Autodesk Fusion 360 part; units mm, degrees
(part 2 of 2)
sketch "Sketch2" plane through (0, 0, 0) normal (0, 1, 0) x (1, 0, 0) in component "Component"
  circle A0 centre (36.4389, -36.7557) radius 32
  line L0 (34.5722, -68.7012) -> (34.5722, -70.4968)
  line L1 (34.5722, -70.4968) -> (36, -73)
  line L2 (36, -73) -> (37, -73)
  line L3 (37, -73) -> (38.5721, -70.4968)
  line L4 (38.5721, -70.4968) -> (38.5721, -68.6845)
  line L5 (43.8241, -69.7477) -> (43.5406, -67.9577)
  line L6 (42.6629, -72.466) -> (43.8241, -69.7477)
  line L7 (41.6753, -72.6224) -> (42.6629, -72.466)
  line L8 (39.8735, -70.3734) -> (41.6753, -72.6224)
  line L9 (39.5926, -68.5999) -> (39.8735, -70.3734)
  line L10 (48.8943, -68.1862) -> (48.3343, -66.4626)
  line L11 (48.1726, -71.0527) -> (48.8943, -68.1862)
  line L12 (47.2216, -71.3617) -> (48.1726, -71.0527)
  line L13 (45.0902, -69.4223) -> (47.2216, -71.3617)
  line L14 (44.5353, -67.7145) -> (45.0902, -69.4223)
  line L15 (53.6578, -65.8508) -> (52.835, -64.236)
  line L16 (53.3934, -68.7949) -> (53.6578, -65.8508)
  line L17 (52.5024, -69.2489) -> (53.3934, -68.7949)
  line L18 (50.0938, -67.6667) -> (52.5024, -69.2489)
  line L19 (49.2786, -66.0668) -> (50.0938, -67.6667)
  line L20 (57.9972, -62.799) -> (56.932, -61.3328)
  line L21 (58.1967, -65.7481) -> (57.9972, -62.799)
  line L22 (57.3877, -66.3359) -> (58.1967, -65.7481)
  line L23 (54.7613, -65.15) -> (57.3877, -66.3359)
  line L24 (53.7058, -63.6974) -> (54.7613, -65.15)
  line L25 (61.8059, -59.1059) -> (60.5244, -57.8244)
  line L26 (62.4642, -61.9875) -> (61.8059, -59.1059)
  line L27 (61.7571, -62.6946) -> (62.4642, -61.9875)
  line L28 (58.9775, -61.9342) -> (61.7571, -62.6946)
  line L29 (57.7078, -60.6645) -> (58.9775, -61.9342)
  line L30 (64.9899, -54.8624) -> (63.5237, -53.7972)
  line L31 (66.0909, -57.6056) -> (64.9899, -54.8624)
  line L32 (65.5031, -58.4146) -> (66.0909, -57.6056)
  line L33 (62.6388, -58.0984) -> (65.5031, -58.4146)
  line L34 (61.1862, -57.043) -> (62.6388, -58.0984)
  line L35 (67.4709, -50.1731) -> (65.8561, -49.3504)
  line L36 (68.9875, -52.7103) -> (67.4709, -50.1731)
  line L37 (68.5335, -53.6013) -> (68.9875, -52.7103)
  line L38 (65.655, -53.7371) -> (68.5335, -53.6013)
  line L39 (64.0551, -52.9219) -> (65.655, -53.7371)
  line L40 (69.1878, -45.1535) -> (67.4642, -44.5934)
  line L41 (71.0826, -47.4222) -> (69.1878, -45.1535)
  line L42 (70.7736, -48.3732) -> (71.0826, -47.4222)
  line L43 (67.9518, -48.9576) -> (70.7736, -48.3732)
  line L44 (66.244, -48.4027) -> (67.9518, -48.9576)
  line L45 (70.0983, -39.927) -> (68.3083, -39.6435)
  line L46 (72.3247, -41.8714) -> (70.0983, -39.927)
  line L47 (72.1683, -42.859) -> (72.3247, -41.8714)
  line L48 (69.4726, -43.8777) -> (72.1683, -42.859)
  line L49 (67.6991, -43.5968) -> (69.4726, -43.8777)
  line L50 (70.18, -34.6225) -> (68.3677, -34.6225)
  line L51 (72.6831, -36.1946) -> (70.18, -34.6225)
  line L52 (72.6831, -37.1946) -> (72.6831, -36.1946)
  line L53 (70.18, -38.6224) -> (72.6831, -37.1946)
  line L54 (68.3844, -38.6224) -> (70.18, -38.6224)
  line L55 (69.4309, -29.3705) -> (67.6409, -29.654)
  line L56 (72.1491, -30.5317) -> (69.4309, -29.3705)
  line L57 (72.3056, -31.5193) -> (72.1491, -30.5317)
  line L58 (70.0566, -33.3211) -> (72.3056, -31.5193)
  line L59 (68.2831, -33.602) -> (70.0566, -33.3211)
  line L60 (67.8694, -24.3003) -> (66.1458, -24.8603)
  line L61 (70.7358, -25.022) -> (67.8694, -24.3003)
  line L62 (71.0448, -25.973) -> (70.7358, -25.022)
  line L63 (69.1054, -28.1044) -> (71.0448, -25.973)
  line L64 (67.3977, -28.6593) -> (69.1054, -28.1044)
  line L65 (65.5339, -19.5368) -> (63.9192, -20.3596)
  line L66 (68.478, -19.8012) -> (65.5339, -19.5368)
  line L67 (68.932, -20.6922) -> (68.478, -19.8012)
  line L68 (67.3499, -23.1008) -> (68.932, -20.6922)
  line L69 (65.75, -23.916) -> (67.3499, -23.1008)
  line L70 (62.4821, -15.1974) -> (61.0159, -16.2626)
  line L71 (65.4313, -14.9979) -> (62.4821, -15.1974)
  line L72 (66.0191, -15.8069) -> (65.4313, -14.9979)
  line L73 (64.8332, -18.4333) -> (66.0191, -15.8069)
  line L74 (63.3805, -19.4888) -> (64.8332, -18.4333)
  line L75 (58.789, -11.3887) -> (57.5075, -12.6702)
  line L76 (61.6707, -10.7304) -> (58.789, -11.3887)
  line L77 (62.3778, -11.4375) -> (61.6707, -10.7304)
  line L78 (61.6173, -14.2171) -> (62.3778, -11.4375)
  line L79 (60.3477, -15.4868) -> (61.6173, -14.2171)
  line L80 (54.5456, -8.2047) -> (53.4803, -9.6709)
  line L81 (57.2888, -7.1037) -> (54.5456, -8.2047)
  line L82 (58.0978, -7.6915) -> (57.2888, -7.1037)
  line L83 (57.7815, -10.5558) -> (58.0978, -7.6915)
  line L84 (56.7261, -12.0084) -> (57.7815, -10.5558)
  line L85 (49.8563, -5.7237) -> (49.0335, -7.3385)
  line L86 (52.3935, -4.2071) -> (49.8563, -5.7237)
  line L87 (53.2845, -4.6611) -> (52.3935, -4.2071)
  line L88 (53.4202, -7.5396) -> (53.2845, -4.6611)
  line L89 (52.605, -9.1395) -> (53.4202, -7.5396)
  line L90 (44.8366, -4.0068) -> (44.2766, -5.7304)
  line L91 (47.1053, -2.112) -> (44.8366, -4.0068)
  line L92 (48.0564, -2.421) -> (47.1053, -2.112)
  line L93 (48.6407, -5.2428) -> (48.0564, -2.421)
  line L94 (48.0858, -6.9506) -> (48.6407, -5.2428)
  line L95 (39.6102, -3.0963) -> (39.3267, -4.8863)
  line L96 (41.5545, -0.8699) -> (39.6102, -3.0963)
  line L97 (42.5422, -1.0263) -> (41.5545, -0.8699)
  line L98 (43.5608, -3.722) -> (42.5422, -1.0263)
  line L99 (43.2799, -5.4955) -> (43.5608, -3.722)
  line L100 (34.3056, -3.0146) -> (34.3056, -4.8269)
  line L101 (35.8777, -0.5115) -> (34.3056, -3.0146)
  line L102 (36.8777, -0.5115) -> (35.8777, -0.5115)
  line L103 (38.3055, -3.0146) -> (36.8777, -0.5115)
  line L104 (38.3055, -4.8102) -> (38.3055, -3.0146)
  line L105 (29.0536, -3.7637) -> (29.3371, -5.5537)
  line L106 (30.2148, -1.0455) -> (29.0536, -3.7637)
  line L107 (31.2025, -0.889) -> (30.2148, -1.0455)
  line L108 (33.0042, -3.138) -> (31.2025, -0.889)
  line L109 (33.2851, -4.9115) -> (33.0042, -3.138)
  line L110 (23.9835, -5.3252) -> (24.5435, -7.0488)
  line L111 (24.7051, -2.4588) -> (23.9835, -5.3252)
  line L112 (25.6562, -2.1498) -> (24.7051, -2.4588)
  line L113 (27.7876, -4.0892) -> (25.6562, -2.1498)
  line L114 (28.3424, -5.7969) -> (27.7876, -4.0892)
  line L115 (19.22, -7.6606) -> (20.0428, -9.2754)
  line L116 (19.4843, -4.7166) -> (19.22, -7.6606)
  line L117 (20.3754, -4.2626) -> (19.4843, -4.7166)
  line L118 (22.7839, -5.8447) -> (20.3754, -4.2626)
  line L119 (23.5991, -7.4446) -> (22.7839, -5.8447)
  line L120 (14.8805, -10.7125) -> (15.9458, -12.1787)
  line L121 (14.6811, -7.7633) -> (14.8805, -10.7125)
  line L122 (15.4901, -7.1755) -> (14.6811, -7.7633)
  line L123 (18.1165, -8.3614) -> (15.4901, -7.1755)
  line L124 (19.1719, -9.8141) -> (18.1165, -8.3614)
  line L125 (11.0719, -14.4056) -> (12.3534, -15.6871)
  line L126 (10.4135, -11.5239) -> (11.0719, -14.4056)
  line L127 (11.1206, -10.8168) -> (10.4135, -11.5239)
  line L128 (13.9002, -11.5773) -> (11.1206, -10.8168)
  line L129 (15.1699, -12.8469) -> (13.9002, -11.5773)
  line L130 (7.8878, -18.649) -> (9.354, -19.7143)
  line L131 (6.7868, -15.9058) -> (7.8878, -18.649)
  line L132 (7.3746, -15.0968) -> (6.7868, -15.9058)
  line L133 (10.2389, -15.4131) -> (7.3746, -15.0968)
  line L134 (11.6916, -16.4685) -> (10.2389, -15.4131)
  line L135 (5.4068, -23.3383) -> (7.0216, -24.1611)
  line L136 (3.8902, -20.8011) -> (5.4068, -23.3383)
  line L137 (4.3442, -19.9101) -> (3.8902, -20.8011)
  line L138 (7.2228, -19.7744) -> (4.3442, -19.9101)
  line L139 (8.8226, -20.5896) -> (7.2228, -19.7744)
  line L140 (3.69, -28.358) -> (5.4136, -28.918)
  line L141 (1.7951, -26.0893) -> (3.69, -28.358)
  line L142 (2.1041, -25.1382) -> (1.7951, -26.0893)
  line L143 (4.926, -24.5539) -> (2.1041, -25.1382)
  line L144 (6.6337, -25.1087) -> (4.926, -24.5539)
  line L145 (2.7795, -33.5844) -> (4.5694, -33.8679)
  line L146 (0.553, -31.6401) -> (2.7795, -33.5844)
  line L147 (0.7095, -30.6524) -> (0.553, -31.6401)
  line L148 (3.4052, -29.6338) -> (0.7095, -30.6524)
  line L149 (5.1787, -29.9147) -> (3.4052, -29.6338)
  line L150 (2.6978, -38.889) -> (4.5101, -38.889)
  line L151 (0.1946, -37.3169) -> (2.6978, -38.889)
  line L152 (0.1946, -36.3169) -> (0.1946, -37.3169)
  line L153 (2.6978, -34.8891) -> (0.1946, -36.3169)
  line L154 (4.4934, -34.8891) -> (2.6978, -34.8891)
  line L155 (3.4469, -44.141) -> (5.2369, -43.8575)
  line L156 (0.7286, -42.9798) -> (3.4469, -44.141)
  line L157 (0.5722, -41.9921) -> (0.7286, -42.9798)
  line L158 (2.8212, -40.1904) -> (0.5722, -41.9921)
  line L159 (4.5947, -39.9095) -> (2.8212, -40.1904)
  line L160 (5.0084, -49.2111) -> (6.732, -48.6511)
  line L161 (2.1419, -48.4895) -> (5.0084, -49.2111)
  line L162 (1.8329, -47.5384) -> (2.1419, -48.4895)
  line L163 (3.7723, -45.407) -> (1.8329, -47.5384)
  line L164 (5.4801, -44.8522) -> (3.7723, -45.407)
  line L165 (7.3438, -53.9746) -> (8.9586, -53.1518)
  line L166 (4.3997, -53.7103) -> (7.3438, -53.9746)
  line L167 (3.9457, -52.8192) -> (4.3997, -53.7103)
  line L168 (5.5279, -50.4107) -> (3.9457, -52.8192)
  line L169 (7.1278, -49.5955) -> (5.5279, -50.4107)
  line L170 (10.3956, -58.3141) -> (11.8618, -57.2488)
  line L171 (7.4465, -58.5135) -> (10.3956, -58.3141)
  line L172 (6.8587, -57.7045) -> (7.4465, -58.5135)
  line L173 (8.0446, -55.0781) -> (6.8587, -57.7045)
  line L174 (9.4972, -54.0227) -> (8.0446, -55.0781)
  line L175 (14.0887, -62.1227) -> (15.3702, -60.8412)
  line L176 (11.2071, -62.7811) -> (14.0887, -62.1227)
  line L177 (10.5, -62.074) -> (11.2071, -62.7811)
  line L178 (11.2604, -59.2944) -> (10.5, -62.074)
  line L179 (12.5301, -58.0247) -> (11.2604, -59.2944)
  line L180 (18.3322, -65.3068) -> (19.3974, -63.8406)
  line L181 (15.589, -66.4078) -> (18.3322, -65.3068)
  line L182 (14.78, -65.82) -> (15.589, -66.4078)
  line L183 (15.0962, -62.9557) -> (14.78, -65.82)
  line L184 (16.1516, -61.503) -> (15.0962, -62.9557)
  line L185 (23.0215, -67.7878) -> (23.8442, -66.173)
  line L186 (20.4843, -69.3044) -> (23.0215, -67.7878)
  line L187 (19.5933, -68.8504) -> (20.4843, -69.3044)
  line L188 (19.4575, -65.9718) -> (19.5933, -68.8504)
  line L189 (20.2727, -64.372) -> (19.4575, -65.9718)
  line L190 (28.0411, -69.5046) -> (28.6012, -67.781)
  line L191 (25.7724, -71.3995) -> (28.0411, -69.5046)
  line L192 (24.8214, -71.0905) -> (25.7724, -71.3995)
  line L193 (24.237, -68.2686) -> (24.8214, -71.0905)
  line L194 (24.7919, -66.5609) -> (24.237, -68.2686)
  line L195 (33.2676, -70.4151) -> (33.5511, -68.6252)
  line L196 (31.3232, -72.6416) -> (33.2676, -70.4151)
  line L197 (30.3355, -72.4851) -> (31.3232, -72.6416)
  line L198 (29.3169, -69.7894) -> (30.3355, -72.4851)
  line L199 (29.5978, -68.0159) -> (29.3169, -69.7894)
  line L200 (36.4389, -36.7557) -> (68.4389, -36.7557) construction
  line L201 (36.4389, -36.7557) -> (36.4389, -68.7557) construction
  circle A1 centre (43.4389, -29.7557) radius 4.19
  circle A2 centre (36.4389, -36.7557) radius 31
  circle A3 centre (43.4389, -57.7557) radius 4.19
  circle A4 centre (43.4389, -43.7557) radius 4.19
  circle A5 centre (29.4389, -43.7557) radius 4.19
  circle A6 centre (29.4389, -29.7557) radius 4.19
  circle A7 centre (29.4389, -57.7557) radius 4.19
  circle A8 centre (15.4389, -43.7557) radius 4.19
  circle A9 centre (57.4389, -43.7557) radius 4.19
  circle A10 centre (57.4389, -29.7557) radius 4.19
  circle A11 centre (15.4389, -29.7557) radius 4.19
  circle A12 centre (29.4389, -15.7557) radius 4.19
  line L202 (36.4389, -36.7557) -> (36.4389, -5.7557) construction
  circle A13 centre (43.4389, -15.7557) radius 4.19
  circle A14 centre (36.4389, -36.7557) radius 22.0695 construction
  arc A15 (38.0191, -58.7686) -> (34.8587, -58.7686) centre (36.4389, -58.8252) ccw
  arc A16 (25.6028, -53.8143) -> (34.8758, -58.5864) centre (29.4389, -57.7557) ccw
  arc A17 (38.002, -58.5864) -> (47.2749, -53.8143) centre (43.4389, -57.7557) ccw
  arc A18 (53.4974, -47.5918) -> (58.2696, -38.3188) centre (57.4389, -43.7557) ccw
  arc A19 (58.4517, -35.1755) -> (58.4517, -38.3359) centre (58.5084, -36.7557) ccw
  arc A20 (58.2696, -35.1926) -> (53.4974, -25.9197) centre (57.4389, -29.7557) ccw
  arc A21 (47.2749, -19.6972) -> (38.002, -14.925) centre (43.4389, -15.7557) ccw
  arc A22 (34.8587, -14.7429) -> (38.0191, -14.7429) centre (36.4389, -14.6862) ccw
  arc A23 (34.8758, -14.925) -> (25.6028, -19.6972) centre (29.4389, -15.7557) ccw
  arc A24 (14.426, -38.3359) -> (14.426, -35.1755) centre (14.3694, -36.7557) ccw
  line L203 (19.3803, -47.5918) -> (25.6028, -53.8143)
  line L204 (47.2749, -53.8143) -> (53.4974, -47.5918)
  line L205 (47.2749, -19.6972) -> (53.4974, -25.9197)
  line L206 (25.6028, -19.6972) -> (19.3803, -25.9197)
  arc A25 (14.6082, -38.3188) -> (19.3803, -47.5918) centre (15.4389, -43.7557) ccw
  arc A26 (16.4435, -39.6879) -> (16.2989, -38.4273) centre (36.4389, -36.7557) ccw construction
  arc A27 (19.3803, -25.9197) -> (14.6082, -35.1926) centre (15.4389, -29.7557) ccw
  line L207 (49.1449, -51.9443) -> (57.0827, -59.8822)
  line L208 (51.7471, -49.3421) -> (59.6778, -57.2728)
  line L209 (51.7471, -24.1694) -> (59.6778, -16.2386)
  line L210 (48.9573, -21.3796) -> (56.8837, -13.4532)
  line L211 (13.15, -16.2953) -> (21.0774, -24.2226)
  line L212 (23.9058, -21.3942) -> (15.9784, -13.4669)
  line L213 (23.9321, -52.1436) -> (16.0065, -60.0692)
  line L214 (21.2453, -49.4568) -> (13.3078, -57.3943)
  line L215 (13.6472, -56.7716) -> (21.4947, -48.9241)
  line L216 (37.6615, -47.5) -> (35.2163, -47.5)
  arc A28 (35.2163, -55) -> (32.2332, -52.0169) centre (32.2332, -55) ccw
  arc A29 (32.2332, -50.4831) -> (35.2163, -47.5) centre (32.2332, -47.5) ccw
  arc A30 (37.6615, -47.5) -> (40.6445, -50.4831) centre (40.6445, -47.5) ccw
  line L217 (40.6445, -55) -> (40.6445, -54.6336)
  line L218 (35.2163, -55) -> (37.6615, -55)
  line L219 (40.2826, -55) -> (40.6445, -55)
  arc A31 (40.6445, -52.0169) -> (37.6615, -55) centre (40.6445, -55) ccw
  line L220 (32.2332, -51.4893) -> (26.2332, -51.4893)
  line L221 (26.2332, -51.4893) -> (26.2332, -51)
  line L222 (26.2332, -51) -> (32.2332, -51)
  line L223 (40.6445, -51.4893) -> (46.6445, -51.4893)
  line L224 (46.6445, -51.4893) -> (46.6445, -51)
  line L225 (46.6445, -51) -> (40.6445, -51)
  line L226 (32.2332, -50.4831) -> (32.2332, -51)
  line L227 (32.2332, -51.4893) -> (32.2332, -52.0169)
  line L228 (40.6445, -52.0169) -> (40.6445, -51.4893)
  line L229 (40.6445, -51) -> (40.6445, -50.4831)
  line L230 (50.1662, -40.9614) -> (50.6831, -40.9614)
  line L231 (50.6831, -46.9614) -> (50.6831, -40.9614)
  arc A32 (47.1831, -35.5331) -> (50.1662, -32.5501) centre (47.1831, -32.5501) ccw
  line L232 (51.7001, -32.5501) -> (51.1725, -32.5501)
  line L233 (51.1725, -32.5501) -> (51.1725, -26.5501)
  line L234 (51.1725, -46.9614) -> (50.6831, -46.9614)
  line L235 (51.1725, -40.9614) -> (51.1725, -46.9614)
  arc A33 (51.7001, -32.5501) -> (54.6831, -35.5331) centre (54.6831, -32.5501) ccw
  line L236 (50.6831, -32.5501) -> (50.1662, -32.5501)
  line L237 (50.6831, -26.5501) -> (50.6831, -32.5501)
  line L238 (47.1831, -35.5331) -> (47.1831, -37.9783)
  arc A34 (50.1662, -40.9614) -> (47.1831, -37.9783) centre (47.1831, -40.9614) ccw
  arc A35 (54.6831, -37.9783) -> (51.7001, -40.9614) centre (54.6831, -40.9614) ccw
  line L239 (51.1725, -40.9614) -> (51.7001, -40.9614)
  line L240 (54.6831, -37.9783) -> (54.6831, -35.5331)
  line L241 (51.1725, -26.5501) -> (50.6831, -26.5501)
  line L242 (40.6445, -23.0284) -> (40.6445, -22.5115)
  line L243 (46.6445, -22.5115) -> (40.6445, -22.5115)
  arc A36 (35.2163, -26.0115) -> (32.2332, -23.0284) centre (32.2332, -26.0115) ccw
  line L244 (32.2332, -21.4945) -> (32.2332, -22.0221)
  line L245 (32.2332, -22.0221) -> (26.2332, -22.0221)
  line L246 (46.6445, -22.0221) -> (46.6445, -22.5115)
  line L247 (40.6445, -22.0221) -> (46.6445, -22.0221)
  arc A37 (32.2332, -21.4945) -> (35.2163, -18.5115) centre (32.2332, -18.5115) ccw
  line L248 (32.2332, -22.5115) -> (32.2332, -23.0284)
  line L249 (26.2332, -22.5115) -> (32.2332, -22.5115)
  line L250 (35.2163, -26.0115) -> (37.6615, -26.0115)
  arc A38 (40.6445, -23.0284) -> (37.6615, -26.0115) centre (40.6445, -26.0115) ccw
  arc A39 (37.6615, -18.5115) -> (40.6445, -21.4945) centre (40.6445, -18.5115) ccw
  line L251 (40.6445, -22.0221) -> (40.6445, -21.4945)
  line L252 (37.6615, -18.5115) -> (35.2163, -18.5115)
  line L253 (26.2332, -22.0221) -> (26.2332, -22.5115)
  line L254 (22.7115, -32.5501) -> (22.1946, -32.5501)
  line L255 (22.1946, -26.5501) -> (22.1946, -32.5501)
  arc A40 (25.6946, -37.9783) -> (22.7115, -40.9614) centre (25.6946, -40.9614) ccw
  line L256 (21.1777, -40.9614) -> (21.7053, -40.9614)
  line L257 (21.7053, -40.9614) -> (21.7053, -46.9614)
  line L258 (21.7053, -26.5501) -> (22.1946, -26.5501)
  line L259 (21.7053, -32.5501) -> (21.7053, -26.5501)
  arc A41 (21.1777, -40.9614) -> (18.1946, -37.9783) centre (18.1946, -40.9614) ccw
  line L260 (22.1946, -40.9614) -> (22.7115, -40.9614)
  line L261 (22.1946, -46.9614) -> (22.1946, -40.9614)
  line L262 (25.6946, -37.9783) -> (25.6946, -35.5331)
  arc A42 (22.7115, -32.5501) -> (25.6946, -35.5331) centre (25.6946, -32.5501) ccw
  arc A43 (18.1946, -35.5331) -> (21.1777, -32.5501) centre (18.1946, -32.5501) ccw
  line L263 (21.7053, -32.5501) -> (21.1777, -32.5501)
  line L264 (18.1946, -35.5331) -> (18.1946, -37.9783)
  line L265 (21.7053, -46.9614) -> (22.1946, -46.9614)
  point P0 (55.8456, -36.2744)
  dimension "d2" = 360
  dimension "d5" = 8.38
  dimension "d6" = 7
  dimension "d7" = 7
  dimension "d8" = 64
  dimension "d9" = 62
  dimension "d10" = 8.38
  dimension "d11" = 7
  dimension "d12" = 14
  dimension "d13" = 8.38
  dimension "d14" = 14
  dimension "d15" = 8.38
  dimension "d16" = 14
  dimension "d17" = 7
  dimension "d18" = 7
  dimension "d19" = 7
  dimension "d20" = 14
  dimension "d21" = 8.38
  dimension "d23" = 14
  dimension "d24" = 8.38
  dimension "d25" = 14
  dimension "d26" = 14
  dimension "d27" = 8.38
  dimension "d29" = 7
  dimension "d30" = 14
  dimension "d31" = 7
  dimension "d32" = 14
  dimension "d33" = 11
  dimension "d34" = 11
  dimension "d35" = 11
  dimension "d36" = 11
  dimension "d37" = 11
  dimension "d38" = 11
  dimension "d39" = 11
  dimension "d40" = 11
  dimension "d41" = 7
  dimension "d42" = 1.5812
  dimension "d43" = 4
  dimension "d44" = 4
  dimension "d45" = 2.4
  dimension "d46" = 2.4
  dimension "d47" = 6
  dimension "d48" = 6
  dimension "d50" = 360
  constraint coincident A0 L0.start
  constraint vertical L0
  constraint horizontal L2
  constraint coincident A0 L4.end
  constraint perpendicular L2 L4
  constraint coincident A0.centre L200.start
  constraint coincident A0 L200.end
  constraint horizontal L200
  constraint coincident A0 L201.end
  constraint perpendicular L200 L201
  constraint concentric A0 A2
  constraint equal A1 A3
  constraint symmetric L200 A1 A4
  constraint symmetric L201 A1 A6
  constraint symmetric L201 A4 A5
  constraint coincident A2 L202.end
  constraint parallel L201 L202
  constraint equal A12 A13
  constraint concentric A7 A16
  constraint concentric A3 A17
  constraint concentric A8 A25
  constraint concentric A11 A27
  constraint concentric A9 A18
  constraint concentric A10 A20
  constraint concentric A13 A21
  constraint concentric A12 A23
  constraint concentric A2 A14
  constraint coincident A14 A15.centre
  constraint coincident L201 A15.centre
  constraint tangent A15 A17
  constraint coincident L200 A19.centre
  constraint coincident A14 A19.centre
  constraint tangent A19 A20
  constraint coincident A14 A22.centre
  constraint coincident L202 A22.centre
  constraint tangent A21 A22
  constraint coincident A14 A24.centre
  constraint tangent A24 A25
  constraint concentric A0 A26
  constraint coincident A14 A15.end
  constraint coincident A14 A15.start
  constraint coincident A16.start A26
  constraint coincident A15 A16.end
  constraint coincident A15 A17.start
  constraint coincident A17.end A26
  constraint coincident A18.start A26
  constraint coincident A14 A19.end
  constraint coincident A14 A19.start
  constraint coincident A19 A18.end
  constraint coincident A20.end A26
  constraint coincident A19 A20.start
  constraint coincident A21.start A26
  constraint coincident A21.end A22
  constraint coincident A14 A22.start
  constraint coincident A14 A22.end
  constraint coincident A23.end A26
  constraint coincident A22 A23.start
  constraint coincident A14 A24.end
  constraint coincident A14 A24.start
  constraint coincident L203.start A26
  constraint coincident L206.end A26
  constraint coincident A8 A26.start
  constraint coincident A24 A25.start
  constraint coincident A24 A27.end
  constraint coincident L204 L207.start
  constraint coincident A2 L207.end
  constraint perpendicular L204 L207
  constraint coincident L204 L208.start
  constraint coincident A2 L208.end
  constraint perpendicular L204 L208
  constraint coincident L205 L209.start
  constraint coincident A2 L209.end
  constraint perpendicular L208 L209
  constraint coincident L205 L210.start
  constraint coincident A2 L210.end
  constraint perpendicular L205 L210
  constraint coincident A2 L211.start
  constraint coincident L206 L211.end
  constraint perpendicular L206 L211
  constraint coincident L206 L212.start
  constraint coincident A2 L212.end
  constraint perpendicular L206 L212
  constraint coincident L203 L213.start
  constraint coincident A2 L213.end
  constraint perpendicular L203 L213
  constraint coincident L203 L214.start
  constraint coincident A2 L214.end
  constraint perpendicular L203 L214
  constraint vertical L217
  constraint horizontal L216
  constraint vertical L226
  constraint coincident A3 L217.end
  constraint collinear L217 L228
  constraint coincident A3 L219.start
  constraint collinear L218 L219
  constraint horizontal L220
  constraint vertical L221
  constraint horizontal L222
  constraint coincident L220.start L226
  constraint horizontal L223
  constraint vertical L224
  constraint horizontal L225
  constraint collinear L226 L227
  constraint collinear L228 L229
  measures "d5" diameter of A3
  measures "d6" distance of L200 A1.centre
  measures "d7" distance of L201 A1.centre
  measures "d8" diameter of A0
  measures "d9" diameter of A2
  measures "d10" diameter of A7
  measures "d11" distance of L201 A7.centre
  measures "d12" distance of A5.centre A7.centre
  measures "d13" diameter of A8
  measures "d14" distance of A5.centre A8.centre
  measures "d15" diameter of A9
  measures "d16" horizontal distance of A4.centre A9.centre
  measures "d17" distance of L200 A9.centre
  measures "d18" distance of L200 A8.centre
  measures "d19" distance of L201 A3.centre
  measures "d20" distance of A3.centre A4.centre
  measures "d21" diameter of A10
  measures "d23" horizontal distance of A1.centre A10.centre
  measures "d24" diameter of A11
  measures "d25" vertical distance of A8.centre A11.centre
  measures "d26" distance of A6.centre A11.centre
  measures "d27" diameter of A12
  measures "d29" distance of A12.centre L202
  measures "d30" distance of A6.centre A12.centre
  measures "d31" distance of L202 A13.centre
  measures "d32" distance of A1.centre A13.centre
  measures "d33" diameter of A16
  measures "d34" diameter of A17
  measures "d35" diameter of A25
  measures "d36" diameter of A27
  measures "d37" diameter of A18
  measures "d38" diameter of A20
  measures "d39" diameter of A21
  measures "d40" diameter of A23
  measures "d41" distance of L200 A10.centre
  measures "d42" radius of A24
  measures "d43" distance of L213 L215
  measures "d44" distance of L211 L212
  measures "d45" distance of L206.end L211.end
  measures "d46" distance of A23.end L212.start
  measures "d47" distance of L221.end L222.end
  measures "d48" distance of L224.end L225.end
extrude "Extrude1" add sketch "Sketch2" along normal mid plane 8 contours A0 | A0 L50 L51 L52 L53 L54 | A0 L55 L56 L57 L58 L59 | A0 L45 L46 L47 L48 L49 | A0 L60 L61 L62 L63 L64 | A0 L40 L41 L42 L43 L44 | A0 L65 L66 L67 L68 L69 | A0 L35 L36 L37 L38 L39 | A0 L70 L71 L72 L73 L74 | A0 L30 L31 L32 L33 L34 | A0 L75 L76 L77 L78 L79 | A0 L25 L26 L27 L28 L29 | A0 L80 L81 L82 L83 L84 | A0 L20 L21 L22 L23 L24 | A0 L85 L86 L87 L88 L89 | A0 L15 L16 L17 L18 L19 | A0 L90 L91 L92 L93 L94 | A0 L10 L11 L12 L13 L14 | A0 L95 L96 L97 L98 L99 | A0 L5 L6 L7 L8 L9 | A0 L100 L101 L102 L103 L104 | A0 L0 L1 L2 L3 L4 | A0 L105 L106 L107 L108 L109 | A0 L195 L196 L197 L198 L199 | A0 L110 L111 L112 L113 L114 | A0 L190 L191 L192 L193 L194 | A0 L115 L116 L117 L118 L119 | A0 L185 L186 L187 L188 L189 | A0 L120 L121 L122 L123 L124 | A0 L180 L181 L182 L183 L184 | A0 L125 L126 L127 L128 L129 | A0 L175 L176 L177 L178 L179 | A0 L130 L131 L132 L133 L134 | A0 L170 L171 L172 L173 L174 | A0 L135 L136 L137 L138 L139 | A0 L165 L166 L167 L168 L169 | A0 L140 L141 L142 L143 L144 | A0 L160 L161 L162 L163 L164 | A0 L145 L146 L147 L148 L149 | A0 L155 L156 L157 L158 L159 | A0 L150 L151 L152 L153 L154 makes body 1 in component "Component"
extrude "Extrude2" add sketch "Sketch2" along normal mid plane 6 separate body contours A2 A18 A19 A20 L204 L205 L208 L209 | A2 A21 A22 A23 L205 L206 L210 L212 | A2 A15 A16 A17 L203 L204 L207 L213 | A2 A24 L203 L206 A25 A27 L211 L214 makes body 2 at (26.2939, 1, 66.0487) makes body 3 at (65.6897, -1, 26.4899) makes body 4 at (12.338, 1, 56.2532) makes body 5 at (39.4021, 1, 5.8977) in component "Component"
extrude "Extrude6" add sketch "Sketch2" along normal mid plane 8 contours A2 L205 L209 L210 | A2 L204 L207 L208 | A15 A16 A17 A18 A19 A20 A21 A22 A23 A24 L203 L204 L205 L206 A25 A27 | A2 L206 L211 L212 | A2 L203 L213 L214 bodies 1 2 3 4 5 in component "Component"
sketch "Sketch3" plane through (0, 0, 0) normal (0, 1, 0) x (-1, 0, 0) in component "Component"
  line L0 (-36.4389, 36.7557) -> (-36.4389, 68.7557)
  line L1 (-32.6946, 35.5331) -> (-32.6946, 37.9783)
  arc A0 (-35.6777, 40.9614) -> (-32.6946, 37.9783) centre (-32.6946, 40.9614) ccw
  arc A1 (-32.6946, 35.5331) -> (-35.6777, 32.5501) centre (-32.6946, 32.5501) ccw
  line L2 (-36.2039, 29.553) -> (-36.2053, 32.5501)
  line L3 (-36.6946, 32.5501) -> (-36.6932, 29.5501)
  arc A2 (-37.2115, 32.5501) -> (-40.1946, 35.5331) centre (-40.1946, 32.5501) ccw
  line L4 (-40.1946, 37.9783) -> (-40.1946, 35.5331)
  arc A3 (-40.1946, 37.9783) -> (-37.2115, 40.9614) centre (-40.1946, 40.9614) ccw
  line L5 (-36.6946, 43.9614) -> (-36.6946, 40.9614)
  line L6 (-36.4389, 46.9614) -> (-36.6946, 46.9614)
  line L7 (-35.6777, 40.9614) -> (-36.2053, 40.9614)
  line L8 (-36.6946, 40.9614) -> (-37.2115, 40.9614)
  line L9 (-37.2115, 32.5501) -> (-36.6946, 32.5501)
  line L10 (-36.2053, 32.5501) -> (-35.6777, 32.5501)
  line L11 (-36.6932, 29.5501) -> (-36.2039, 29.553)
  line L12 (-36.2053, 40.9614) -> (-36.2053, 43.9614)
  line L13 (-36.2053, 43.9614) -> (-36.6946, 43.9614)
  line L14 (-36.6946, 43.9614) -> (-36.6946, 40.9614)
  dimension "d67" = 3
  constraint vertical L12
  constraint horizontal L13
  constraint vertical L14
  constraint coincident L0 L6.start
  measures "d67" distance of L3.start L3.end
extrude "Extrude8" cut sketch "Sketch3" along normal blind 4 and the other way blind 4 bodies 1 in component "Component"
sketch "Sketch2 (2)" plane through (0, 0, 0) normal (0, 1, 0) x (-1, 0, 0)
extrude "Extrude7" [suppressed] in component "Component"
component "Component" placed x (1, 0, 0) y (0, 1, 0) z (0, 0, 1) at (0, 0, 0)
equation "d5 = ( 4.19 * 2 ) * 1 mm"
